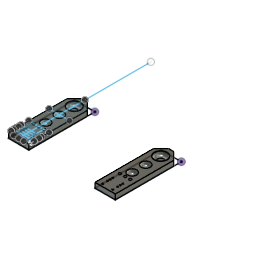
test1 (Autodesk Fusion 360 design; units mm, degrees)
part number: 2026-04-22-15-27-53-499
part number: 2026-04-22-15-33-21-274
Autodesk Fusion 360 part; units mm, degrees
sketch "Esquisse1" plane through (0, 0, 0) normal (0, 0, 1) x (1, 0, 0) in component "Component"
  line L0 (0, 0) -> (-80, 0)
  line L1 (-80, 0) -> (-80, -260)
  line L2 (-80, -260) -> (0, -260)
  line L3 (0, -260) -> (0, 0)
  dimension "d2" = 80
  dimension "d3" = 260
  constraint horizontal L0
  constraint vertical L1
  constraint horizontal L2
  constraint vertical L3
  constraint coincident L0.start L3.end
  measures "d2" distance of L0.start L0.end
  measures "d3" distance of L0.start L2.end
extrude "Extrusion1" add sketch "Esquisse1" along normal blind 20 in component "Component"
hole "Perçage1" at (-40.5158, -41.0549, 20) direction (0, 0, -1) diameter 50 depth 15 tip angle 180 in component "Component"
sketch "Esquisse1 (2)" plane through (0, 0, 20) normal (0, 0, 1) x (-1, 0, 0)
  circle A0 centre (40.5158, 41.0549) radius 25
  line L0 (0, 260) -> (0, 0)
  line L1 (0, 0) -> (80, 0)
  line L2 (80, 0) -> (80, 260)
  line L3 (80, 260) -> (0, 260)
  line L4 (40, -260) -> (40, 260)
  line L5 (0, 100.1565) -> (80, 100.1565)
  line L6 (0, 180.5797) -> (80, 180.5797)
  line L7 (20.3399, 260) -> (20.3399, 180.5797)
  line L8 (59.7707, 260) -> (59.7707, 180.5797)
  line L9 (0, 210.2505) -> (80, 210.2505)
  line L10 (0, 230.5515) -> (80, 230.5515)
  line L11 (0, 220.0106) -> (80, 220.0106)
  line L12 (0, 239.9212) -> (80, 239.9212)
  line L13 (0, 249.6813) -> (80, 249.6813)
  point P0 (40, 0)
  constraint midpoint L4 P0
  constraint coincident L1 P0
  constraint coincident L3 L4.end
  constraint perpendicular L3 L4
  constraint coincident L0 L5.start
  constraint coincident L2 L5.end
  constraint perpendicular L2 L5
  constraint coincident L0 L6.start
  constraint coincident L2 L6.end
  constraint perpendicular L2 L6
  constraint coincident L3 L7.start
  constraint coincident L6 L7.end
  constraint perpendicular L6 L7
  constraint coincident L3 L8.start
  constraint coincident L6 L8.end
  constraint perpendicular L6 L8
  constraint coincident L0 L9.start
  constraint coincident L2 L9.end
  constraint perpendicular L2 L9
  constraint coincident L0 L10.start
  constraint coincident L2 L10.end
  constraint perpendicular L2 L10
  constraint coincident L0 L11.start
  constraint coincident L2 L11.end
  constraint perpendicular L2 L11
  constraint coincident L0 L12.start
  constraint coincident L2 L12.end
  constraint perpendicular L2 L12
  constraint coincident L2 L13.end
  constraint perpendicular L2 L13
hole "Perçage2" at (-40.2505, -100.1565, 20) direction (0, 0, -1) diameter 35 depth 15 tip angle 180 in component "Component"
hole "Perçage3" at (-40.2505, -153.2515, 20) direction (0, 0, -1) diameter 35 depth 15 tip angle 180 in component "Component"
hole "Perçage4" at (-20.3399, -180.5797, 20) direction (0, 0, -1) diameter 10 depth 15 tip angle 180 in component "Component"
hole "Perçage5" at (-40.1512, -180.6942, 20) direction (0, 0, -1) diameter 10 depth 15 tip angle 180 in component "Component"
hole "Perçage6" at (-60.0584, -181.372, 20) direction (0, 0, -1) diameter 10 depth 15 tip angle 180 in component "Component"
hole "Perçage7" at (-20.4915, -210.1519, 20) direction (0, 0, -1) diameter 6 depth 15 tip angle 180 in component "Component"
hole "Perçage8" at (-59.96, -210.0461, 20) direction (0, 0, -1) diameter 6 depth 15 tip angle 180 in component "Component"
sketch "Esquisse2" plane through (0, 0, 20) normal (0, 0, 1) x (-1, 0, 0)
  point P0 (20.3408, 220.1831)
  point P1 (59.7814, 220.1831)
  point P2 (59.7814, 249.7814)
  point P3 (20.3408, 249.7814)
  point P4 (20.3408, 230.5042)
  point P5 (59.7814, 230.5042)
hole "Perçage9" at (-20.3408, -220.1831, 20) at (-20.3408, -230.5042, 20) at (-20.3408, -249.7814, 20) at (-59.7814, -249.7814, 20) at (-59.7814, -230.5042, 20) at (-59.7814, -220.1831, 20) direction (0, 0, -1) diameter 6 depth 10 tip angle 180 in component "Component"
chamfer "Chanfrein1" distance 30 angle 45 1 edges at (-80, 0, 10) measured on face at (-26.6667, 0, 6.6667) in component "Component"
chamfer "Chanfrein2" distance 30 angle 45 1 edges at (0, 0, 10) measured on face at (0, -173.3333, 13.3333) in component "Component"
fillet "Congé1" chord length 20 1 edges at (-63.824, -32.0145, 5) in component "Component"
fillet "Congé2" radius 15 1 edges at (-56.5663, -93.8282, 5) in component "Component"
fillet "Congé3" radius 15 1 edges at (-56.5663, -146.9232, 5) in component "Component"
component "Component" placed x (1, 0, 0) y (0, 1, 0) z (0, 0, 1) at (0, 0, 0)
component "Component" placed x (1, 0, 0) y (0, 1, 0) z (0, 0, 1) at (340, 0, 0)
